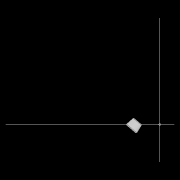
# Autodesk Inventor part: Rollers_Rotor_TSB
Saved by Autodesk Inventor 2022.2 (Build 262287010, 287A)
## iProperties
Created: 2022-05-21
Part Number: Rollers_Rotor_TSB
Material: Generic
Document SubType Name: Modeling
Designer: Árni Þór Þorgeirsson
Density: 1 g/cm^3
Appearance: Default
Author: Árni Þór Þorgeirsson
Autodesk Inventor part; units mm, degrees
ref_plane "YZ Plane" through (0, 0, 0) normal (1, 0, 0) x (0, 1, 0)
ref_plane "XZ Plane" through (0, 0, 0) normal (0, 1, 0) x (-1, 0, 0)
ref_plane "XY Plane" through (0, 0, 0) normal (0, 0, 1) x (1, 0, 0)
sketch "Sketch1" plane through (0, 0, 0) normal (0, 0, 1) x (1, 0, 0)
  circle A0 centre (0, 0) radius 14.029612 construction
  line L0 (0, 0) -> (14.029612, 0)
  line L1 (0, 0) -> (14.029612, 4.025)
  line L2 (14.029612, 0) -> (14.029612, 4.025)
  circle A1 centre (0, 0) radius 55.5
  dimension "d56" = 14.02961
  dimension "d57" = 4.025
  dimension "d400" = 55.5
  dimension "d403" = 2.75
  dimension "d404" = 1.5
  dimension "d412" = 5.4
  dimension "d427" = 1.5
  dimension "d428" = 1.5
  dimension "d429" = 5.4
  dimension "d430" = 5.4
  dimension "d435" = 30
  constraints: 40 end point, 8 coincident, 3 centre point, 2 horizontal alignment, 1 horizontal, 1 point on line, 46 other
  measures "d428" radius of A0
sketch "Sketch7" plane through (0, 0, 0) normal (0, 1, 0) x (-1, 0, 0)
  line L0 (0, 0) -> (0, 16.473921)
  line L1 (0, 0) -> (-14.029612, 0) construction
  line L2 (0, 16.473921) -> (-14.029612, 0) construction
  line L3 (0, 16.473921) -> (-19.349377, 0) construction
  line L4 (0, 16.473921) -> (-13.18191, -5.250938) construction
  line L5 (0, 0) -> (0, -16.473921)
  line L6 (0, -16.473921) -> (-14.029612, 0) construction
  line L7 (0, -16.473921) -> (-19.349377, 0) construction
  line L8 (0, -16.473921) -> (-13.18191, 5.250938) construction
  line L9 (-13.18191, 5.250938) -> (-19.349377, 0) construction
  line L10 (-9.995818, 0) -> (-19.211561, -7.846217) construction
  line L11 (-9.995818, 0) -> (-18.326933, 7.093051) construction
  line L12 (0, -30.378651) -> (0, 66.954459)
  line L13 (-55.5, -5.99191) -> (-55.5, 6.008042)
  line L14 (15.727341, 0) -> (-94.364044, 0)
  line L15 (-16.689131, 2.264915) -> (-11.370092, -2.264915) construction
  line L16 (-11.370092, 2.264915) -> (-16.689131, -2.264915) construction
  line L17 (-26.151002, -15.930308) -> (-40.378296, -15.930308) construction
  line L18 (-40.378296, -15.930308) -> (-40.378296, -12.753867) construction
  line L19 (-40.378296, -12.753867) -> (-26.151002, -12.753867) construction
  line L20 (-26.151002, -12.753867) -> (-26.151002, -15.930308) construction
  point P0 (-55.5, 0)
  dimension "Roller_Side_difference" = -0.015
  dimension "d90" = 16.47392
  dimension "d201" = 55.5
  dimension "d343" = 99.1629
  dimension "d344" = 99.1783
  dimension "d367" = 8.1
  constraints: 28 end point, 9 point on line, 3 midpoint, 3 vertical, 2 horizontal, 2 parallel, 2 perpendicular, 1 collinear, 1 symmetric about line, 2 other
  measures "d90" distance of L0.start L0.end
  measures "d201" distance between parallel lines of L5 L13
  measures "d343" angle of L10 L8
  measures "d344" angle of L7 L10
  measures "d367" distance of L3.end L8.end
sketch "Roller1" plane through (0, 0, 0) normal (0, 1, 0) x (-1, 0, 0)
  line L0 (0, 16.473921) -> (-13.18191, -5.250938) construction
  line L1 (0, 16.473921) -> (-19.349377, 0) construction
  line L2 (-9.995818, 0) -> (-18.326933, 7.093051) construction
  line L3 (0, -16.473921) -> (-19.349377, 0) construction
  line L4 (-10.067645, -0.070182) -> (-13.148647, -5.147923)
  line L5 (-13.148647, -5.147923) -> (-19.252966, 0.04925)
  line L6 (-19.252966, 0.04925) -> (-14.730445, 3.899692)
  line L7 (-14.730445, 3.899692) -> (-10.067645, -0.070182)
  line L8 (-12.404416, 1.919328) -> (-16.20556, -2.545289)
  line L9 (-11.643, 1.271065) -> (-15.444144, -3.193553)
  point P0 (0, 0)
  point P1 (-16.200806, -2.549337)
  dimension "d345" = 0.025
  dimension "d346" = 0.025
  dimension "d347" = 0.1
  dimension "d348" = 0.1
  dimension "d349" = 99.1783
  dimension "d350" = 99.1629
  dimension "d357" = 1
  dimension "d369" = 4.01478
  constraints: 12 end point, 5 parallel, 4 point on line, 1 midpoint, 1 perpendicular
  measures "d345" distance between parallel lines of L0 L4
  measures "d346" distance between parallel lines of L1 L6
  measures "d347" distance between parallel lines of L3 L5
  measures "d348" distance between parallel lines of L2 L7
  measures "d349" angle of L6 L7
  measures "d350" angle of L4 L7
  measures "d357" distance between parallel lines of L8 L9
  measures "d369" distance from line of L4.end L8
sketch "Roller2" plane through (0, 0, 0) normal (0, 1, 0) x (-1, 0, 0)
  line L0 (0, -16.473921) -> (-13.18191, 5.250938) construction
  line L1 (-9.995818, 0) -> (-19.211561, -7.846217) construction
  line L2 (0, -16.473921) -> (-19.349377, 0) construction
  line L3 (0, 16.473921) -> (-19.349377, 0) construction
  line L4 (-13.148647, 5.147923) -> (-10.067645, 0.070182)
  line L5 (-10.067645, 0.070182) -> (-14.730445, -3.899692)
  line L6 (-14.730445, -3.899692) -> (-19.252966, -0.04925)
  line L7 (-19.252966, -0.04925) -> (-13.148647, 5.147923)
  line L8 (-16.200806, 2.549337) -> (-12.399663, -1.915281)
  line L9 (-15.439391, 3.1976) -> (-11.638247, -1.267018)
  point P0 (0, 0)
  dimension "d351" = 0.025
  dimension "d352" = 0.025
  dimension "d354" = 0.1
  dimension "d355" = 99.1629
  dimension "d356" = 99.1783
  dimension "d370" = 0.1
  dimension "d371" = 1
  constraints: 12 end point, 5 parallel, 3 point on line, 1 midpoint, 1 perpendicular
  measures "d351" distance between parallel lines of L0 L4
  measures "d352" distance between parallel lines of L2 L6
  measures "d354" distance between parallel lines of L1 L5
  measures "d355" angle of L5 L4
  measures "d356" angle of L6 L5
  measures "d370" distance from line of L3 L8.start
  measures "d371" distance between parallel lines of L9 L8
sketch "Sketch22" plane through (0, 0, 0) normal (0, 1, 0) x (-1, 0, 0)
  line L0 (-31.75595, 8.021531) -> (-17.528657, 8.021531) construction
  line L1 (-17.528657, 8.021531) -> (-17.528657, 4.84509) construction
  line L2 (-17.528657, 4.84509) -> (-31.75595, 4.84509) construction
  line L3 (-31.75595, 4.84509) -> (-31.75595, 8.021531) construction
  point P0 (0, 0)
  dimension "Roller_Side_difference" = -0.015
  constraints: 2 other
sketch "Sketch2" plane through (0, 0, 0) normal (0, 1, 0) x (-1, 0, 0)
  line L0 (0, 0) -> (0, 14.029612) construction
  line L1 (0, 0) -> (-14.029612, 0)
  line L2 (0, 0) -> (0, -14.029612)
  line L3 (0, -14.029612) -> (-14.029612, 0) construction
  line L4 (0, 14.029612) -> (-14.029612, 0) construction
  line L5 (-78.636704, 53.049729) -> (0, 14.029612) construction
  line L6 (-34.829637, 15.681058) -> (0, 14.029612) construction
  line L7 (-34.829637, 15.681058) -> (0, -14.029612) construction
  line L8 (-48.318301, 16.320622) -> (0, -14.029612) construction
  point P0 (-17.81718, -3.787568)
  constraints: 16 end point, 3 point on line, 1 perpendicular, 1 symmetric about line, 1 vertical
sketch "Sketch23" plane through (0, 0, 0) normal (0, 1, 0) x (-1, 0, 0)
  line L0 (0, -16.473921) -> (-13.18191, 5.250938) construction
  line L1 (0, -16.473921) -> (-19.349377, 0) construction
  line L2 (0, 16.473921) -> (-13.18191, -5.250938) construction
  line L3 (-13.18191, 5.250938) -> (-19.349377, 0) construction
  line L4 (0, 16.473921) -> (-19.349377, 0) construction
  line L5 (-13.18191, 5.250938) -> (-13.18191, -5.250938) construction
  line L6 (15.727341, 0) -> (-94.364044, 0)
  line L7 (-12.154792, 3.750938) -> (-9.910325, 0.051874)
  line L8 (-9.910325, -0.051874) -> (-12.154792, -3.750938)
  line L9 (-15.097987, 3.750938) -> (-19.414204, 0.076142)
  line L10 (-19.414204, -0.076142) -> (-15.097987, -3.750938)
  arc A0 (-19.414204, 0.076142) -> (-19.414204, -0.076142) centre (-19.349377, 0) ccw
  arc A1 (-9.910325, -0.051874) -> (-9.910325, 0.051874) centre (-9.995818, 0) ccw
  line L11 (-12.154792, 3.750938) -> (-12.154792, 5.250938)
  line L12 (-12.154792, 5.250938) -> (-1, 5.250938)
  line L13 (-1, 5.250938) -> (-1, -5.250938)
  line L14 (-1, -5.250938) -> (-12.154792, -5.250938)
  line L15 (-12.154792, -5.250938) -> (-12.154792, -3.750938)
  line L16 (-15.097987, 3.750938) -> (-15.097987, 5.250938)
  line L17 (-15.097987, 5.250938) -> (-55.5, 5.250938)
  line L18 (-55.5, 5.250938) -> (-55.5, -5.250938)
  line L19 (-15.097987, -3.750938) -> (-15.097987, -5.250938)
  line L20 (-15.097987, -5.250938) -> (-55.5, -5.250938)
  line L21 (-13.18191, 5.250938) -> (-13.18191, 5.250938)
  line L22 (-13.18191, -5.250938) -> (-13.18191, -5.250938)
  line L23 (0, -30.378651) -> (0, 66.954459)
  line L24 (-19.503636, 0) -> (-55.5, 0)
  point P0 (0, 0)
  point P1 (-9.87885, 0)
  point P2 (-19.449377, 0)
  point P3 (-55.5, 0)
  dimension "d378" = 90
  dimension "d379" = 0.1
  dimension "d380" = 0.1
  dimension "d381" = 0.1
  dimension "d382" = 0.1
  dimension "d383" = 0.1
  dimension "d384" = 10.502
  dimension "d385" = 0
  dimension "d386" = 0
  dimension "d391" = 1
  dimension "d392" = 55.5
  dimension "d393" = 1.5
  dimension "d394" = 1.5
  dimension "d395" = 1.5
  dimension "d396" = 1.5
  constraints: 36 end point, 10 point on line, 9 vertical, 4 horizontal, 4 parallel, 4 point on circle, 4 tangent, 2 centre point, 1 equal radius, 1 midpoint
  measures "d378" angle of L6 L5
  measures "d379" radius of A0
  measures "d380" distance between parallel lines of L9 L4
  measures "d381" distance between parallel lines of L10 L1
  measures "d382" distance between parallel lines of L0 L7
  measures "d383" distance between parallel lines of L2 L8
  measures "d385" distance of L2.end L22.end
  measures "d386" distance of L0.end L21.end
  measures "d391" distance between parallel lines of L23 L13
  measures "d392" distance between parallel lines of L18 L23
  measures "d393" distance of L9.start L16.end
  measures "d394" distance of L7.start L11.end
  measures "d395" distance of L14.end L8.end
  measures "d396" distance of L10.end L19.end
revolve "RevRoller1" add sketch "Roller1" angle 360 about axis through (12.404416, 0, 1.919328) along (0.6482639, 0, -0.7614157) contours L4 L5 L9 L7
fillet "Fillet1" radius 0.5 2 edges at (14.7412, 0, 3.9088) (19.2625, 0, 0.0573)
sketch "Sketch26" plane through (0, 0, 5.251) normal (0, 0, 1) x (1, 0, 0)
  arc A0 (-55.47973, 1.499863) -> (-55.47973, -1.499863) centre (-55.5, 0) ccw
  line L0 (-58.2, 1.558846) -> (-55.5, 3.117691)
  line L1 (-55.5, 3.117691) -> (-52.8, 1.558846)
  line L2 (-52.8, 1.558846) -> (-52.8, -1.558846)
  line L3 (-52.8, -1.558846) -> (-55.5, -3.117691)
  line L4 (-55.5, -3.117691) -> (-58.2, -1.558846)
  line L5 (-58.2, -1.558846) -> (-58.2, 1.558846)
  circle A1 centre (0, 0) radius 55.5
  point P0 (-55.415099, -3.068674)
  point P1 (-55.415099, 3.068674)
  dimension "d417" = 5.4
  dimension "d472" = 1.5
  constraints: 1 centre point, 1 coincident, 2 other
  measures "d472" radius of A1
sketch "Sketch14" plane through (0, 0, -6) normal (0, 0, -1) x (-1, 0, 0)
  spline S0 degree 3 poles (-56.8, 0) (-56.8, -1.431881) (-57.026593, -2.821774) (-57.314092, -4.037688) (-57.767634, -5.955845) (-58.324925, -7.569677) (-58.722177, -9.395339) (-59.136874, -11.301177) (-59.386946, -13.435019) (-59.224701, -15.723511) (-59.041721, -18.304483) (-58.301884, -21.037122) (-57.069228, -23.431656) (-55.971572, -25.563942) (-54.514733, -27.402841) (-52.991577, -28.859445) (-51.609846, -30.180803) (-50.199133, -31.18712) (-48.777188, -32.156453) (-47.658195, -32.919264) (-46.48864, -33.676075) (-45.287633, -34.714466) (-44.246149, -35.614932) (-43.223884, -36.761375) (-42.446498, -37.948052) (-41.552186, -39.313219) (-40.961475, -40.639527) (-40.402311, -41.881595) (-39.698144, -43.445755) (-39.012013, -44.971422) (-38.036421, -46.541904) (-36.852293, -48.44808) (-35.229027, -50.390903) (-33.172449, -51.991109) (-31.082785, -53.617058) (-28.576167, -54.843072) (-26.098683, -55.508164) (-23.966746, -56.080492) (-21.888687, -56.253442) (-19.99643, -56.216327) (-18.226323, -56.181608) (-16.627473, -55.964803) (-14.870408, -55.813491) (-13.64371, -55.707852) (-12.286984, -55.640346) (-10.841781, -55.797651) (-9.405099, -55.954028) (-7.958194, -56.356058) (-6.72296, -56.840927) (-4.720046, -57.627134) (-3.160865, -58.523891) (-1.374264, -59.285893) (0.43393, -60.057105) (2.484074, -60.721054) (4.785864, -61.008032) (7.29738, -61.321158) (10.069876, -61.145772) (12.636394, -60.427936) (15.068469, -59.747703) (17.276682, -58.604718) (19.078145, -57.306263) (20.675036, -56.155257) (21.947787, -54.911578) (23.179094, -53.650366) (24.093052, -52.71421) (25.006164, -51.733074) (26.173802, -50.758008) (27.251307, -49.858209) (28.581523, -49.007828) (29.920293, -48.422475) (31.362039, -47.792099) (32.729271, -47.438027) (34.006062, -47.112779) (35.709882, -46.67875) (37.357471, -46.274501) (39.106618, -45.584899) (41.122062, -44.79031) (43.245842, -43.605028) (45.144764, -41.957103) (47.125697, -40.238007) (48.812365, -38.031705) (49.948214, -35.729443) (50.978693, -33.640754) (51.562264, -31.514277) (51.875473, -29.551465) (52.163791, -27.744649) (52.224462, -26.087015) (52.389409, -24.26927) (52.500122, -23.049187) (52.674768, -21.705521) (53.082371, -20.317797) (53.486023, -18.943526) (54.125098, -17.604696) (54.807763, -16.484696) (55.88488, -14.717543) (56.994603, -13.378644) (58.020634, -11.829602) (59.057735, -10.263846) (60.042061, -8.478079) (60.746022, -6.391794) (61.563199, -3.969975) (61.952412, -1.167763) (61.739294, 1.551053) (61.547741, 3.994746) (60.885294, 6.331699) (59.984948, 8.322377) (59.176867, 10.109055) (58.203586, 11.60696) (57.20438, 13.015762) (56.346663, 14.225075) (55.431932, 15.394279) (54.571362, 16.88266) (53.894644, 18.053065) (53.296047, 19.449594) (52.941401, 20.830246) (52.552633, 22.343737) (52.424689, 23.753818) (52.324012, 25.055013) (52.184403, 26.859393) (52.085193, 28.576265) (51.714961, 30.452969) (51.28784, 32.618042) (50.483443, 34.970332) (49.158524, 37.176656) (47.799936, 39.439045) (45.903076, 41.493315) (43.816379, 43.014429) (41.987076, 44.347912) (40.049977, 45.272999) (38.218731, 45.915148) (36.450804, 46.535094) (34.796175, 46.888834) (33.001138, 47.375434) (31.816009, 47.696699) (30.521309, 48.102017) (29.224612, 48.747174) (27.936085, 49.388266) (26.725059, 50.259376) (25.737673, 51.133196) (24.124849, 52.560519) (22.965436, 53.937323) (21.542494, 55.265954) (20.138156, 56.577215) (18.481715, 57.869905) (16.475722, 58.911451) (14.165758, 60.110822) (11.411802, 60.921686) (8.673039, 61.114083) (6.216698, 61.286639) (3.815099, 60.974418) (1.724855, 60.389113) (-0.129049, 59.869988) (-1.725431, 59.159596) (-3.275956, 58.416395) (-4.506134, 57.826744) (-5.740001, 57.188084) (-7.231871, 56.648969) (-8.509412, 56.187305) (-9.992918, 55.847926) (-11.410335, 55.746452) (-12.986274, 55.633629) (-14.405683, 55.762793) (-15.720374, 55.893001) (-17.512575, 56.070502) (-19.228258, 56.26353) (-21.14738, 56.213015) (-23.35139, 56.155001) (-25.800578, 55.754238) (-28.188185, 54.822549) (-30.641265, 53.865311) (-32.975397, 52.347878) (-34.818644, 50.559208) (-36.474242, 48.952631) (-37.727206, 47.167636) (-38.679148, 45.444153) (-39.602271, 43.772847) (-40.235424, 42.170761) (-41.073244, 40.426521) (-41.604313, 39.3209) (-42.257018, 38.118991) (-43.132465, 36.982168) (-43.986349, 35.873347) (-45.02128, 34.895963) (-46.014928, 34.116317) (-47.65816, 32.826989) (-49.178947, 31.937998) (-50.701661, 30.79158) (-52.259778, 29.618509) (-53.844584, 28.184055) (-55.231092, 26.35155) (-56.798454, 24.280015) (-58.054532, 21.711787) (-58.70314, 19.059492) (-59.291585, 16.653218) (-59.385373, 14.222627) (-59.157392, 12.057591) (-58.957075, 10.155262) (-58.529173, 8.473739) (-58.065474, 6.821513) (-57.71572, 5.575291) (-57.32751, 4.313182) (-57.062989, 2.838558) (-56.903092, 1.947178) (-56.8, 0.977593) (-56.8, 0) knots 0 0 0 0 3.63018867 3.63018867 3.63018867 9.35696823 9.35696823 9.35696823 15.33524763 15.33524763 15.33524763 22.07757634 22.07757634 22.07757634 28.08148705 28.08148705 28.08148705 33.52793428 33.52793428 33.52793428 37.81399081 37.81399081 37.81399081 41.53075392 41.53075392 41.53075392 45.80655899 45.80655899 45.80655899 51.19116605 51.19116605 51.19116605 57.72674671 57.72674671 57.72674671 64.36747302 64.36747302 64.36747302 70.08198523 70.08198523 70.08198523 75.42761126 75.42761126 75.42761126 79.15966987 79.15966987 79.15966987 82.86972023 82.86972023 82.86972023 88.88550846 88.88550846 88.88550846 94.97400254 94.97400254 94.97400254 101.61724685 101.61724685 101.61724685 107.91249493 107.91249493 107.91249493 113.49286598 113.49286598 113.49286598 117.63499042 117.63499042 117.63499042 121.45737705 121.45737705 121.45737705 125.57377362 125.57377362 125.57377362 131.06691996 131.06691996 131.06691996 137.39636219 137.39636219 137.39636219 143.99916005 143.99916005 143.99916005 149.98943627 149.98943627 149.98943627 155.50363213 155.50363213 155.50363213 159.20479832 159.20479832 159.20479832 162.87008171 162.87008171 162.87008171 168.65322103 168.65322103 168.65322103 174.49875886 174.49875886 174.49875886 181.28442381 181.28442381 181.28442381 187.38343345 187.38343345 187.38343345 192.85743132 192.85743132 192.85743132 197.55629967 197.55629967 197.55629967 201.25130677 201.25130677 201.25130677 205.3018314 205.3018314 205.3018314 210.91872996 210.91872996 210.91872996 217.39870578 217.39870578 217.39870578 224.04334598 224.04334598 224.04334598 229.86836977 229.86836977 229.86836977 235.49198409 235.49198409 235.49198409 239.20483501 239.20483501 239.20483501 242.89429398 242.89429398 242.89429398 248.92075827 248.92075827 248.92075827 254.86843 254.86843 254.86843 261.71735865 261.71735865 261.71735865 267.86002373 267.86002373 267.86002373 273.30815026 273.30815026 273.30815026 277.63066309 277.63066309 277.63066309 281.33218517 281.33218517 281.33218517 285.4476808 285.4476808 285.4476808 291.0579716 291.0579716 291.0579716 297.50109046 297.50109046 297.50109046 304.12089172 304.12089172 304.12089172 310.06677175 310.06677175 310.06677175 315.83264406 315.83264406 315.83264406 319.48745935 319.48745935 319.48745935 323.05225137 323.05225137 323.05225137 328.94747413 328.94747413 328.94747413 334.9797604 334.9797604 334.9797604 341.79888944 341.79888944 341.79888944 347.98549115 347.98549115 347.98549115 353.42140754 353.42140754 353.42140754 357.52154898 357.52154898 357.52154898 360 360 360 360
  circle A0 centre (0, 0) radius 55.5
  point P0 (-56.8, 0)
  dimension "d226" = 5.4
  dimension "d277" = 76.5
  dimension "d319" = 30
  dimension "d320" = 5.4
  dimension "d321" = 5.4
  dimension "d246" = 2.75
  dimension "d254" = 2.75
  dimension "d255" = 3
  dimension "d293" = 60
  dimension "d294" = 90
  dimension "d305" = 30
  dimension "d107" = 0.05
  dimension "d108" = 0.05
  dimension "d109" = 0.05
  dimension "d110" = 0.05
  dimension "d112" = 0.5
  dimension "d113" = 0.5
  dimension "d114" = 0.5
  dimension "d115" = 83.9087
  dimension "d116" = 83.6941
  dimension "d117" = 1
  dimension "d118" = 0.05
  dimension "d119" = 0.05
  dimension "d120" = 0.05
  dimension "d121" = 0.05
  dimension "d122" = 0.5
  dimension "d123" = 0.5
  dimension "d124" = 83.9087
  dimension "d125" = 83.6941
  dimension "d126" = 1
  dimension "d39" = 0.05
  dimension "d41" = 0.05
  dimension "d42" = 0.5
  dimension "d43" = 0.5
  dimension "d44" = 0.5
  dimension "d45" = 0.5
  dimension "d46" = 0.5
  dimension "d47" = 0.5
  dimension "d48" = 2
  dimension "d16" = 0.05
  dimension "d17" = 0.05
  dimension "d18" = 0.05
  dimension "d19" = 0.5
  dimension "d20" = 0.5
  dimension "d21" = 0.5
  dimension "d22" = 0.5
  dimension "d23" = 0.5
  dimension "d24" = 0.5
  dimension "d28" = 2
  constraints: 8 end point, 4 point on circle, 3 parallel, 3 tangent, 2 centre point, 3 other
equation "\"Roller_Side_difference\" = -0.015459deg"
equation "\"Roller_Hole_Radius\" = 1"
equation "\"Distance_To_Bearing\" = 21.63839"
body "Solid1"
body "Solid2"
body "Solid3"
body "Solid4"
body "Solid5"
